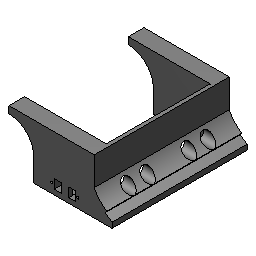
Zumo alejo v2 (Autodesk Fusion 360 design; units mm, degrees)
Autodesk Fusion 360 part; units mm, degrees
note: some values were not read from the file. Set by a fixed rule: which sketch regions a step uses.
sketch "Boceto1" plane through (0, 0, 0) normal (0, 0, 1) x (1, 0, 0)
  line L0 (0, 0) -> (200, 0)
  line L1 (200, 0) -> (200, 200)
  line L2 (200, 200) -> (0, 200)
  line L3 (0, 200) -> (0, 0)
  line L4 (5, 5) -> (195, 5)
  line L5 (195, 5) -> (195, 195)
  line L6 (195, 195) -> (5, 195)
  line L7 (5, 195) -> (5, 5)
  line L8 (195, 100) -> (5, 100)
  dimension "d1" = 200
  dimension "d2" = 200
  dimension "d3" = 190
  dimension "d4" = 190
  constraint horizontal L0
  constraint vertical L1
  constraint horizontal L2
  constraint vertical L3
  constraint coincident L0.start L3.end
  constraint horizontal L4
  constraint vertical L5
  constraint horizontal L6
  constraint vertical L7
  constraint midpoint L5 L8.start
  constraint midpoint L7 L8.end
  measures "d1" distance of L0.start L0.end
  measures "d2" distance of L0.start L2.end
  measures "d3" distance of L4.start L4.end
  measures "d4" distance of L4.start L6.end
sketch "Boceto2" plane through (0, 0, 0) normal (0, 1, 0) x (1, 0, 0)
  line L0 (5, 0) -> (195, 0)
  line L1 (195, 0) -> (195, -80)
  line L2 (195, -80) -> (5, -80)
  line L3 (5, -80) -> (5, 0)
  line L4 (5, 0) -> (75, 0)
  line L5 (40, 0) -> (40, -70)
  circle A0 centre (40, -29.8581) radius 30
  line L6 (40, -70) -> (40, -80)
  line L7 (58.6, 54.5) -> (58.6, 67.5)
  line L8 (43.85, 54.5) -> (54.3, 54.5)
  line L9 (77.1, 54.5) -> (77.1, 67.5)
  line L10 (40.1, 64.75) -> (43.85, 64.75)
  circle A1 centre (77.1, 61) radius 3.75
  line L11 (43.85, 67.5) -> (43.85, 54.5)
  line L12 (64.35, 54.5) -> (64.35, 67.5)
  line L13 (54.3, 67.5) -> (43.85, 67.5)
  circle A2 centre (40.1, 61) radius 3.75
  line L14 (73.35, 67.5) -> (73.35, 54.5)
  line L15 (73.35, 54.5) -> (64.35, 54.5)
  line L16 (77.1, 64.75) -> (73.35, 64.75)
  line L17 (40.1, 57.25) -> (43.85, 57.25)
  line L18 (73.35, 67.5) -> (73.35, 54.5)
  line L19 (40.1, 67.5) -> (40.1, 54.5)
  line L20 (77.1, 57.25) -> (73.35, 57.25)
  line L21 (43.85, 67.5) -> (43.85, 54.5)
  line L22 (77.1, 67.5) -> (40.1, 67.5)
  line L23 (73.35, 67.5) -> (43.85, 67.5)
  circle A3 centre (40.1, 61) radius 1.6
  circle A4 centre (77.1, 61) radius 1.6
  line L24 (54.3, 54.5) -> (54.3, 67.5)
  line L25 (73.35, 67.5) -> (73.35, 54.5)
  line L26 (77.1, 54.5) -> (40.1, 54.5)
  line L27 (73.35, 54.5) -> (64.35, 54.5)
  line L28 (64.35, 67.5) -> (73.35, 67.5)
  line L29 (100, -10) -> (137, -10)
  line L30 (137, -10) -> (137, -23)
  line L31 (137, -23) -> (100, -23)
  line L32 (100, -23) -> (100, -10)
  line L33 (185, 0) -> (185, -80)
  line L34 (200, 0) -> (185, -10.5031)
  line L35 (200, 0) -> (218.3116, 0) construction
  line L36 (200, 0) -> (175.4254, -17.2073)
  line L37 (175.4254, -17.2073) -> (175.4254, 0)
  line L38 (80, -3) -> (185, -3)
  line L39 (175.4254, -17.2073) -> (177.1462, -19.6647)
  line L40 (177.1462, -19.6647) -> (177.3608, -19.9713)
  line L41 (177.3608, -19.9713) -> (179.5533, -18.436)
  line L42 (160, -60) -> (160, -80)
  arc A5 (177.3608, -19.9713) -> (160, -40) centre (208.604, -64.5912) ccw
  line L43 (160, -60) -> (160, -40)
  circle A6 centre (40, -35) radius 35
  line L44 (75, 0) -> (75, -35)
  line L45 (80, -3) -> (75, -3)
  line L46 (160, -40) -> (160, -3)
  line L47 (155, -80) -> (155, -3)
  dimension "d5" = 190
  dimension "d6" = 80
  dimension "d7" = 70
  dimension "d9" = 70
  dimension "d10" = 60
  dimension "d58" = 37
  dimension "d59" = 13
  dimension "d60" = 29.5
  dimension "d61" = 3.2
  dimension "d63" = 13
  dimension "d64" = 9
  dimension "d65" = 10.45
  dimension "d19" = 37
  dimension "d20" = 13
  dimension "d21" = 145
  dimension "d22" = 30
  dimension "d29" = 3
  dimension "d30" = 70
  constraint horizontal L0
  constraint vertical L1
  constraint horizontal L2
  constraint vertical L3
  constraint perpendicular L3 L4
  constraint midpoint L4 L5.start
  constraint perpendicular L4 L5
  constraint coincident L5 A0.centre
  constraint coincident L2 L6.end
  constraint perpendicular L2 L6
  constraint midpoint A1.centre L9
  constraint midpoint A2.centre L19
  constraint perpendicular L19 L26
  constraint coincident L8.start L26
  constraint perpendicular L21 L26
  constraint perpendicular L19 L22
  constraint coincident L13.start L22
  constraint concentric A1 A4
  constraint coincident L16.start A1
  constraint coincident L16.start L9
  constraint coincident L16.end L14
  constraint tangent A1 L16
  constraint perpendicular L14 L16
  constraint coincident L20.start A1
  constraint coincident L20.start L9
  constraint coincident L20.end L25
  constraint tangent A1 L20
  constraint perpendicular L20 L25
  constraint concentric A2 A3
  constraint tangent L11 A2
  constraint coincident L17.start A2
  constraint coincident L17.start L19
  constraint coincident L17.end L11
  constraint tangent A2 L17
  constraint coincident L10.start L19
  constraint coincident L10.start A2
  constraint coincident L10.end L21
  constraint tangent L10 A2
  constraint horizontal L29
  constraint vertical L30
  constraint horizontal L31
  constraint vertical L32
  constraint coincident L0 L33.start
  constraint perpendicular L0 L33
  constraint horizontal L35
  constraint coincident L33 L34.end
  constraint parallel L34 L36
  constraint coincident L0 L37.end
  constraint perpendicular L0 L37
  constraint coincident L33 L38.end
  constraint perpendicular L33 L38
  constraint perpendicular L36 L39
  constraint parallel L39 L40
  constraint perpendicular L39 L41
  constraint coincident L2 L42.end
  constraint perpendicular L2 L42
  constraint tangent L41 A5
  constraint parallel L42 L43
  constraint midpoint L5 A6.centre
  constraint coincident A6 L44.end
  constraint tangent A6 L44
  constraint coincident L44 L45.end
  constraint perpendicular L44 L45
  constraint coincident L38 L46.end
  constraint perpendicular L38 L46
  constraint coincident L38 L47.end
  constraint perpendicular L38 L47
  constraint coincident L2 L47.start
  measures "d5" distance of L0.start L0.end
  measures "d6" distance of L0.start L2.end
  measures "d7" distance of L0.start L4.end
  measures "d9" distance of L5.start L5.end
  measures "d10" diameter of A0
  measures "d58" distance of L19.start L9.end
  measures "d59" distance of L9.end L9.start
  measures "d60" distance of L11.start L14.start
  measures "d61" diameter of A4
  measures "d63" distance of L14.end L14.start
  measures "d64" distance of L12.start L14.end
  measures "d65" distance of L8.end L8.start
  measures "d19" distance of L29.start L29.end
  measures "d20" distance of L29.start L31.end
  measures "d21" angle of L34 L35
  measures "d22" distance of L34.start L36.end
  measures "d29" distance of L36.end L39.end
  measures "d30" diameter of A6
sketch "Boceto4" plane through (185, 0, 0) normal (1, 0, 0) x (0, 1, 0)
  line L0 (52.5, 38) -> (52.5, 18)
  line L1 (30, 38) -> (75, 38)
  line L2 (190, 80) -> (0, 80)
  line L3 (52.5, 18) -> (32.5, 18)
  line L4 (24, 3) -> (24, 10.5031)
  line L5 (0, 16) -> (95, 16)
  line L6 (24, 10.5031) -> (0, 10.5031)
  line L7 (95, 16) -> (95, 40)
  line L8 (0, 80) -> (0, 0)
  line L9 (0, 3) -> (24, 3)
  line L10 (0, 16) -> (0, 40)
  line L11 (75, 18) -> (30, 18)
  line L12 (52.5, 28) -> (39, 28)
  line L13 (190, 0) -> (190, 80)
  line L14 (75, 38) -> (75, 18)
  circle A0 centre (66, 28) radius 8
  line L15 (95, 80) -> (95, 0)
  line L16 (95, 30) -> (95, 50.6611)
  line L17 (0, 40) -> (0, 16)
  line L18 (32.5, 18) -> (32.5, 20.5)
  line L19 (30, 18) -> (30, 38)
  circle A1 centre (39, 28) radius 8
  circle A2 centre (32.5, 20.5) radius 1
  line L20 (0, 0) -> (190, 0)
  line L21 (95, 40) -> (0, 40)
  line L22 (0, 10.5031) -> (0, 3)
  dimension "d39" = 190
  dimension "d40" = 80
  dimension "d41" = 45
  dimension "d42" = 20
  dimension "d43" = 20
  dimension "d44" = 2.5
  dimension "d45" = 2
  dimension "d46" = 13.5
  dimension "d47" = 16
  constraint horizontal L20
  constraint vertical L13
  constraint horizontal L2
  constraint vertical L8
  constraint coincident L8.end L20.start
  constraint midpoint L15.start L2
  constraint midpoint L15.end L20
  constraint horizontal L21
  constraint vertical L17
  constraint horizontal L5
  constraint vertical L7
  constraint coincident L5.start L8
  constraint midpoint L7.end L15
  constraint vertical L16
  constraint coincident L16.end L15
  constraint horizontal L1
  constraint vertical L14
  constraint horizontal L11
  constraint vertical L19
  constraint midpoint L0.start L1
  constraint perpendicular L0 L1
  constraint perpendicular L0 L3
  constraint perpendicular L11 L18
  constraint coincident L18.end A2.centre
  constraint midpoint L12.start L0
  constraint perpendicular L0 L12
  constraint coincident L12.end A1.centre
  constraint symmetric L0 A0 A1
  measures "d39" distance of L13.start L8.end
  measures "d40" distance of L2.end L8.end
  measures "d41" distance of L1.start L1.end
  measures "d42" distance of L1.start L11.end
  measures "d43" distance of L3.end L0.end
  measures "d44" distance of L3.end L18.end
  measures "d45" diameter of A2
  measures "d46" distance of L12.start L12.end
  measures "d47" diameter of A1
extrude "Extruir2" add sketch "Boceto2" along normal blind 95 contours L33 L36 L37 L38 | L37 L38 L39 L40 A5 L46 | L2 L38 L42 L43 L46 L47 makes body 1
extrude "Extruir3" add sketch "Boceto2" along normal blind 22 separate body contours L2 L6 L38 A6 L44 L45 L47 | L29 L30 L31 L32 makes body 2
extrude "Extruir4" cut sketch "Boceto4" against normal blind 30 contours A0 | A1 bodies 1
extrude "Extruir5" add sketch "Boceto2" along normal blind 7.2 separate body contours L7 L22 L23 L24 L26 | L7 L12 L22 L23 L26 | L12 L14 L15 L18 L22 L23 L25 L26 L27 L28 | L8 L11 L13 L21 L22 L23 L24 L26 | A1 L14 L18 L20 L25 | L11 A2 L17 L21 | A1 L14 L16 L18 L25 | L10 L11 A2 L21 | L9 A1 A4 | L9 A1 A4 | A2 L19 A3 | A2 L19 A3 | L9 A4 | L9 A4 | L19 A3 | L19 A3 makes body 3
extrude "Extruir6" add sketch "Boceto2" against normal blind 15 contours L12 L14 L15 L18 L22 L23 L25 L26 L27 L28 | L8 L11 L13 L21 L22 L23 L24 L26 | L9 A4 | L9 A4 | L19 A3 | L19 A3 bodies 3
extrude "Extruir7" add sketch "Boceto2" against normal blind 9 contours L7 L22 L23 L24 L26 | L7 L12 L22 L23 L26 bodies 3
move_body "Desplazar1" bodies 3 to x (1, 0, 0) y (0, 1, 0) z (0, 0, 1) at (59.9, 14.8, 77.5)
combine "Combinar1" operation cut target body 2 tool bodies 3
move_body "Desplazar2" bodies 2 1 to x (1, 0, 0) y (0, 1, 0) z (0, 0, 1) at (0, 5, 0)
sketch "Boceto5" plane through (0, 0, 0) normal (0, 0, 1) x (1, 0, 0)
  line L0 (155, 27) -> (162.5, 27)
  line L1 (170, 27) -> (170, 12)
  line L2 (170, 12) -> (155, 12)
  line L3 (155, 12) -> (155, 27)
  line L4 (170, 12) -> (162.5, 12)
  line L5 (162.5, 12) -> (162.5, 19.5)
  line L6 (162.5, 19.5) -> (170, 19.5)
  line L7 (170, 19.5) -> (170, 12)
  line L8 (162.5, 27) -> (155, 27)
  line L9 (155, 27) -> (155, 34)
  line L10 (155, 34) -> (170, 34)
  line L11 (170, 34) -> (170, 27)
  line L12 (162.5, 19.5) -> (162.5, 27)
  line L13 (185, 5) -> (40, 5)
  line L14 (40, 5) -> (40, 100)
  line L15 (40, 100) -> (185, 100)
  line L16 (185, 100) -> (185, 5)
  line L17 (113, 27) -> (107, 27)
  line L18 (107, 27) -> (107, 33)
  line L19 (107, 33) -> (113, 33)
  line L20 (113, 33) -> (113, 27)
  circle A0 centre (110, 30) radius 1.5
  dimension "d70" = 7.5
  dimension "d75" = 145
  dimension "d76" = 95
  dimension "d77" = 6
  dimension "d78" = 6
  dimension "d79" = 3
  constraint horizontal L0
  constraint vertical L1
  constraint horizontal L2
  constraint vertical L3
  constraint horizontal L4
  constraint vertical L5
  constraint horizontal L6
  constraint vertical L7
  constraint horizontal L8
  constraint vertical L9
  constraint horizontal L10
  constraint vertical L11
  constraint horizontal L13
  constraint vertical L14
  constraint horizontal L15
  constraint vertical L16
  constraint horizontal L17
  constraint vertical L18
  constraint horizontal L19
  constraint vertical L20
  measures "d70" distance of L1.end L4.end
  measures "d75" distance of L13.start L13.end
  measures "d76" distance of L13.start L15.end
  measures "d77" distance of L17.start L17.end
  measures "d78" distance of L17.start L19.end
  measures "d79" diameter of A0
extrude "Extruir8" add sketch "Boceto5" along normal blind 12 separate body contours L1 L2 L4 L5 L6 L7 makes body 4
extrude "Extruir9" add sketch "Boceto5" along normal blind 3 separate body contours L0 L1 L6 L8 L9 L10 L11 L12 makes body 5
move_body "Desplazar3" bodies 5 to x (1, 0, 0) y (0, 1, 0) z (0, 0, 1) at (0, 0, 9)
combine "Combinar2" operation add target body 4 tool bodies 5
combine "Combinar3" operation cut target body 1 tool bodies 4
extrude "Extruir10" add sketch "Boceto5" along normal blind 3 separate body contours L17 L18 L19 L20 makes body 6
copy_body "CopiarPegarCuerpos1" bodies 6 makes body 7
move_body "Desplazar4" bodies 7 to x (1, 0, 0) y (0, 1, 0) z (0, 0, 1) at (-20, 0, 3)
move_body "Desplazar5" bodies 6 to x (1, 0, 0) y (0, 1, 0) z (0, 0, 1) at (42, 22.5, 3)
combine "Combinar4" operation add target body 1 tool bodies 2 7 6
mirror "Simetría2" about plane through (0, 100, 0) normal (0, 1, 0) of bodies 1 merged
move_body "Desplazar6" bodies 1 to x (1, 0, 0) y (0, 1, 0) z (0, 0, 1) at (0, 0, -3)
equation "d54 = 21.6 mm - 14.4 mm"
